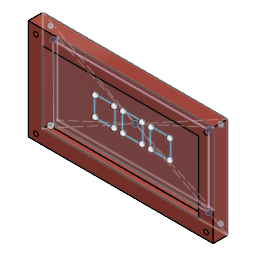
Macropad (Autodesk Fusion 360 design; units mm, degrees)
part number: 2026-06-07-03-08-04-925
Autodesk Fusion 360 part; units mm, degrees
sketch "Sketch4" plane through (0, 0, 0) normal (0, 0, 1) x (1, 0, 0)
  line L0 (53.2905, 24.45) -> (-53.2905, 24.45)
  line L1 (-53.2905, 24.45) -> (-53.2905, -24.45)
  line L2 (-53.2905, -24.45) -> (53.2905, -24.45)
  line L3 (53.2905, -24.45) -> (53.2905, 24.45)
  line L4 (53.2905, 24.45) -> (-53.2905, -24.45) construction
  line L5 (-53.2905, 24.45) -> (53.2905, -24.45) construction
  line L6 (-63.2905, -34.45) -> (63.2905, -34.45)
  line L7 (63.2905, -34.45) -> (63.2905, 34.45)
  line L8 (63.2905, 34.45) -> (-63.2905, 34.45)
  line L9 (-63.2905, 34.45) -> (-63.2905, -34.45)
  line L10 (-63.2905, -34.45) -> (63.2905, 34.45) construction
  line L11 (63.2905, -34.45) -> (-63.2905, 34.45) construction
  circle A0 centre (-58, 29) radius 1.45
  circle A1 centre (-58, -30) radius 1.45
  circle A2 centre (58.5, 29) radius 1.45
  circle A3 centre (58.5, -30) radius 1.45
  point P0 (-58, -30)
  dimension "d20" = 10
  dimension "d21" = 10
  dimension "d22" = 10
  dimension "d23" = 10
  dimension "d24" = 48.9
  dimension "d25" = 106.581
  dimension "d26" = 126.581
  dimension "d27" = 68.9
  dimension "d34" = 2.9
  dimension "d38" = 2.9
  dimension "d39" = 2.9
  dimension "d40" = 2.9
  constraint horizontal L0
  constraint perpendicular L0 L1
  constraint parallel L0 L2
  constraint parallel L1 L3
  constraint coincident L4 origin
  constraint coincident L5 origin
  constraint horizontal L6
  constraint perpendicular L6 L7
  constraint parallel L6 L8
  constraint parallel L7 L9
  constraint coincident L10 origin
  constraint coincident L11 origin
  measures "d20" distance of L0.start L7
  measures "d21" distance of L2.end L6
  measures "d22" distance of L0.end L8
  measures "d23" distance of L1.end L9
  measures "d24" distance of L0.start L2.end
  measures "d25" distance of L0.start L0.end
  measures "d26" distance of L7.end L8.end
  measures "d27" distance of L6.end L7.end
  measures "d34" diameter of A0
  measures "d38" diameter of A1
  measures "d39" diameter of A2
  measures "d40" diameter of A3
extrude "Extrude1" add sketch "Sketch4" along normal blind 3 contours L0 L1 L2 L3
extrude "Extrude2" add sketch "Sketch4" along normal blind 10 contours L6 L7 L8 L9 | A0 | A1 | A2 | A3
extrude "Extrude3" cut sketch "Sketch4" along normal blind 14 contours A0
extrude "Extrude4" cut sketch "Sketch4" along normal blind 14 contours A1
extrude "Extrude5" cut sketch "Sketch4" along normal blind 14 contours A3
extrude "Extrude6" cut sketch "Sketch4" along normal blind 14 contours A2
sketch "plate-2026-06-09T10_15_21.263Z" plane through (0, 0, 3) normal (0, 0, 1) x (1, 0, 0)
  line L0 (-24.2585, 6.9573) -> (-11.2585, 6.9573)
  line L1 (-24.2585, -7.0427) -> (-11.2585, -7.0427)
  line L2 (-24.7585, 6.4573) -> (-24.7585, -6.5427)
  line L3 (-10.7585, 6.4573) -> (-10.7585, -6.5427)
  arc A0 (-24.2585, 6.9573) -> (-24.7585, 6.4573) centre (-24.2585, 6.4573) ccw
  arc A1 (-10.7585, 6.4573) -> (-11.2585, 6.9573) centre (-11.2585, 6.4573) ccw
  arc A2 (-24.7585, -6.5427) -> (-24.2585, -7.0427) centre (-24.2585, -6.5427) ccw
  arc A3 (-11.2585, -7.0427) -> (-10.7585, -6.5427) centre (-11.2585, -6.5427) ccw
  line L4 (-5.2085, 6.9573) -> (7.7915, 6.9573)
  line L5 (-5.2085, -7.0427) -> (7.7915, -7.0427)
  line L6 (-5.7085, 6.4573) -> (-5.7085, -6.5427)
  line L7 (8.2915, 6.4573) -> (8.2915, -6.5427)
  arc A4 (-5.2085, 6.9573) -> (-5.7085, 6.4573) centre (-5.2085, 6.4573) ccw
  arc A5 (8.2915, 6.4573) -> (7.7915, 6.9573) centre (7.7915, 6.4573) ccw
  arc A6 (-5.7085, -6.5427) -> (-5.2085, -7.0427) centre (-5.2085, -6.5427) ccw
  arc A7 (7.7915, -7.0427) -> (8.2915, -6.5427) centre (7.7915, -6.5427) ccw
  line L8 (13.8415, 6.9573) -> (26.8415, 6.9573)
  line L9 (13.8415, -7.0427) -> (26.8415, -7.0427)
  line L10 (13.3415, 6.4573) -> (13.3415, -6.5427)
  line L11 (27.3415, 6.4573) -> (27.3415, -6.5427)
  arc A8 (13.8415, 6.9573) -> (13.3415, 6.4573) centre (13.8415, 6.4573) ccw
  arc A9 (27.3415, 6.4573) -> (26.8415, 6.9573) centre (26.8415, 6.4573) ccw
  arc A10 (13.3415, -6.5427) -> (13.8415, -7.0427) centre (13.8415, -6.5427) ccw
  arc A11 (26.8415, -7.0427) -> (27.3415, -6.5427) centre (26.8415, -6.5427) ccw
  line L12 (-53, -25) -> (53.2905, -24.45)
  line L13 (-53.2905, 24.45) -> (53.2905, 24.45)
  line L14 (-53, -25) -> (-53.2905, 24.45)
  line L15 (53.2905, -24.45) -> (53.2905, 24.45)
  line L16 (53.2905, -24.45) -> (53.2905, 24.45)
  line L17 (53.2905, 24.45) -> (-53.2905, 24.45)
  dimension "d65" = 13
  dimension "d66" = 13
  dimension "d67" = 13
  dimension "d68" = 13
  dimension "d69" = 13
  dimension "d70" = 13
  dimension "d71" = 49.45
  dimension "d72" = 106.2905
  constraint coincident L13.end L15.end
  constraint coincident L13.start L14.end
  constraint coincident L12.end L15.start
  measures "d65" distance of A0.centre A1.centre
  measures "d66" distance of A0.centre A2.centre
  measures "d67" distance of A4.centre A5.centre
  measures "d68" distance of A4.centre A6.centre
  measures "d69" distance of A8.centre A9.centre
  measures "d70" distance of A8.centre A10.centre
  measures "d71" vertical distance of L12.start L13.start
  measures "d72" horizontal distance of L12.start L12.end
extrude "Extrude7" add sketch "plate-2026-06-09T10_15_21.263Z" along normal blind 3
extrude "Extrude8" cut sketch "plate-2026-06-09T10_15_21.263Z" along normal blind 3
